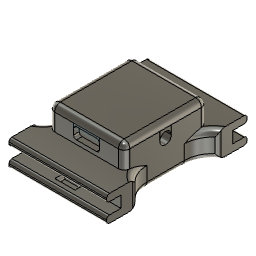
Tremolometer case (Autodesk Fusion 360 design; units mm, degrees)
Autodesk Fusion 360 part; units mm, degrees
sketch "Sketch1" plane through (0, 0, 0) normal (0, 0, 1) x (1, 0, 0)
  line L0 (0, 0) -> (26.2, 0)
  line L1 (26.2, 0) -> (26.2, 28.9)
  line L2 (26.2, 28.9) -> (0, 28.9)
  line L3 (0, 28.9) -> (0, 0)
  dimension "d4" = 26.2
  dimension "d5" = 28.9
  constraint horizontal L0
  constraint vertical L1
  constraint horizontal L2
  constraint vertical L3
  constraint coincident L0.start L3.end
  measures "d4" distance of L0.start L0.end
  measures "d5" distance of L0.start L2.end
extrude "Extrude1" add sketch "Sketch1" along normal blind 15 makes body 1
sketch "Sketch2" plane through (0, 0, 15) normal (0, 0, 1) x (-1, 0, 0)
  line L0 (-4, -24.9) -> (-22.2, -24.9)
  line L1 (-22.2, -24.9) -> (-22.2, -2)
  line L2 (-22.2, -2) -> (-4, -2)
  line L3 (-4, -2) -> (-4, -24.9)
  line L4 (0, -28.9) -> (0, 0)
  line L5 (-26.2, -28.9) -> (0, -28.9)
  line L6 (-26.2, 0) -> (-26.2, -28.9)
  line L7 (0, 0) -> (-26.2, 0)
  dimension "d9" = 4
  dimension "d10" = 4
  dimension "d11" = 4
  dimension "d12" = 2
  constraint horizontal L0
  constraint vertical L1
  constraint horizontal L2
  measures "d9" distance of L3 L4
  measures "d10" distance of L0 L5
  measures "d11" distance of L1 L6
  measures "d12" distance of L2 L7
extrude "Extrude2" cut sketch "Sketch2" against normal blind 6 contours L0 L1 L2 L3 bodies 1
sketch "Sketch4" plane through (0, 0, 0) normal (0, -1, 0) x (1, 0, 0)
  line L0 (0, 0) -> (26.2, 0)
  line L1 (26.2, 0) -> (26.2, 15)
  line L2 (26.2, 15) -> (0, 15)
  line L3 (0, 15) -> (0, 0)
  line L4 (9.6, 10.38) -> (16.6, 10.38)
  line L5 (17.6, 11.38) -> (17.6, 13.38)
  line L6 (16.6, 14.38) -> (9.6, 14.38)
  line L7 (8.6, 13.38) -> (8.6, 11.38)
  arc A0 (9.6, 14.38) -> (8.6, 13.38) centre (9.6, 13.38) ccw
  arc A1 (17.6, 13.38) -> (16.6, 14.38) centre (16.6, 13.38) ccw
  arc A2 (16.6, 10.38) -> (17.6, 11.38) centre (16.6, 11.38) ccw
  arc A3 (8.6, 11.38) -> (9.6, 10.38) centre (9.6, 11.38) ccw
  point P0 (8.6, 10.38)
  point P1 (17.6, 10.38)
  point P2 (8.6, 14.38)
  dimension "d26" = 9
  dimension "d27" = 4
  dimension "d28" = 1
  dimension "d29" = 1
  dimension "d30" = 1
  dimension "d31" = 1
  dimension "d32" = 0.62
  dimension "d33" = 8.6
  constraint horizontal L4
  constraint vertical L5
  constraint horizontal L6
  constraint vertical L7
  constraint coincident P2 L6
  constraint coincident P2 L7
  constraint tangent L6 A0
  constraint tangent L7 A0
  constraint tangent L6 A1
  constraint tangent L5 A1
  constraint coincident P1 L5
  constraint coincident P1 L4
  constraint tangent L5 A2
  constraint tangent L4 A2
  constraint coincident P0 L7
  constraint coincident P0 L4
  constraint tangent L7 A3
  constraint tangent L4 A3
  measures "d26" distance of P0 P1
  measures "d27" distance of P0 P2
  measures "d28" radius of A0
  measures "d29" radius of A1
  measures "d30" radius of A2
  measures "d31" radius of A3
  measures "d32" distance of L2 L6
  measures "d33" distance of L1 L5
extrude "Extrude3" cut sketch "Sketch4" against normal blind 6 contours L4 L5 L6 L7 A0 A1 A2 A3 bodies 1
sketch "Sketch5" plane through (26.2, 0, 0) normal (1, 0, 0) x (0, 1, 0)
  line L0 (0, 0) -> (28.9, 0)
  line L1 (28.9, 0) -> (28.9, 15)
  line L2 (28.9, 15) -> (0, 15)
  line L3 (0, 15) -> (0, 0)
  circle A0 centre (14.45, 12) radius 2
  dimension "d37" = 4
  dimension "d38" = 14.45
  dimension "d39" = 3
  measures "d37" diameter of A0
  measures "d38" distance of L3 A0.centre
  measures "d39" distance of L2 A0.centre
extrude "Extrude4" cut sketch "Sketch5" against normal blind 8.5 contours A0 bodies 1
sketch "Sketch9" plane through (0, 0, 15) normal (0, 0, 1) x (-1, 0, 0)
  line L0 (-22.2, -24.9) -> (-22.2, -2)
  line L1 (-22.2, -2) -> (-4, -2)
  line L2 (-4, -2) -> (-4, -24.9)
  line L3 (-4, -24.9) -> (-22.2, -24.9)
  line L4 (0, -28.9) -> (0, 0)
  line L5 (0, 0) -> (-26.2, 0)
  line L6 (-26.2, 0) -> (-26.2, -28.9)
  line L7 (-26.2, -28.9) -> (0, -28.9)
  line L8 (-2, -26.9) -> (-24.2, -26.9)
  line L9 (-24.2, -26.9) -> (-24.2, -2)
  line L10 (-24.2, -2) -> (-2, -2)
  line L11 (-2, -2) -> (-2, -26.9)
  dimension "d71" = 2
  dimension "d72" = 2
  dimension "d73" = 2
  dimension "d74" = 2
  constraint horizontal L8
  constraint vertical L9
  constraint horizontal L10
  constraint vertical L11
  measures "d71" distance of L5 L10
  measures "d72" distance of L6 L9
  measures "d73" distance of L4 L11
  measures "d74" distance of L7 L8
extrude "Extrude8" add sketch "Sketch9" along normal blind 1 contours L0 L2 L3 L8 L9 L10 L11 bodies 1
extrude "Extrude9" add 1 faces at (10.0667, 0.6667, 15) along direction (0, 0, 1) blind 2 separate body on bodies 1 makes body 2
sketch "Sketch10" plane through (0, 26.9, 0) normal (0, -1, 0) x (1, 0, 0)
  line L0 (2, 15) -> (24.2, 15)
  line L1 (24.2, 15) -> (24.2, 17)
  line L2 (24.2, 17) -> (2, 17)
  line L3 (2, 17) -> (2, 15)
  line L4 (2, 17) -> (26.2, 17)
  line L5 (26.2, 17) -> (26.2, 16)
  line L6 (26.2, 16) -> (2, 16)
  line L7 (2, 16) -> (2, 17)
  dimension "d82" = 24.2
  dimension "d83" = 1
  constraint horizontal L4
  constraint vertical L5
  constraint horizontal L6
  constraint vertical L7
  constraint coincident L2.end L3.start
  measures "d82" distance of L2.end L4.end
  measures "d83" distance of L2.end L6.end
extrude "Extrude10" add sketch "Sketch10" along normal blind 26.9 contours L1 L4 L5 L6 bodies 2
sketch "Sketch19" plane through (0, 0, 0) normal (0, -1, 0) x (1, 0, 0)
  line L0 (16.6, 10.38) -> (9.6, 10.38)
  arc A0 (8.6, 11.38) -> (9.6, 10.38) centre (9.6, 11.38) ccw
  line L1 (8.6, 11.38) -> (8.6, 13.38)
  arc A1 (9.6, 14.38) -> (8.6, 13.38) centre (9.6, 13.38) ccw
  line L2 (9.6, 14.38) -> (16.6, 14.38)
  arc A2 (17.6, 13.38) -> (16.6, 14.38) centre (16.6, 13.38) ccw
  line L3 (17.6, 13.38) -> (17.6, 11.38)
  arc A3 (16.6, 10.38) -> (17.6, 11.38) centre (16.6, 11.38) ccw
  line L4 (0, 0) -> (26.2, 0)
  line L5 (26.2, 0) -> (26.2, 15)
  line L6 (26.2, 15) -> (0, 15)
  line L7 (0, 15) -> (0, 0)
  line L8 (0, 0) -> (26.2, 0)
  line L9 (26.2, 0) -> (26.2, 9)
  line L10 (26.2, 9) -> (0, 9)
  line L11 (0, 9) -> (0, 0)
  dimension "d170" = 26.2
  dimension "d171" = 9
  constraint horizontal L8
  constraint vertical L9
  constraint horizontal L10
  constraint vertical L11
  constraint coincident L4.start L7.end
  measures "d170" distance of L4.start L4.end
  measures "d171" distance of L4.start L10.end
extrude "Extrude19" add sketch "Sketch19" along normal blind 10 contours L4 L5 L7 L8 L9 L10 L11 bodies 1
sketch "Sketch20" plane through (26.2, 0, 0) normal (1, 0, 0) x (0, 1, 0)
  circle A0 centre (14.45, 12) radius 2
  line L0 (-10, 0) -> (28.9, 0)
  line L1 (28.9, 0) -> (28.9, 15)
  line L2 (28.9, 15) -> (0, 15)
  line L3 (0, 15) -> (0, 9)
  line L4 (0, 9) -> (-10, 9)
  line L5 (-10, 9) -> (-10, 0)
  line L6 (-10, 9) -> (0, 9)
  line L7 (0, 9) -> (0, 0)
  line L8 (0, 0) -> (-10, 0)
  line L9 (-10, 0) -> (-10, 9)
  dimension "d174" = 10
  dimension "d175" = 9
  constraint horizontal L6
  constraint vertical L7
  constraint horizontal L8
  constraint vertical L9
  constraint coincident L4.end L5.start
  measures "d174" distance of L4.end L3.end
  measures "d175" distance of L4.end L0.start
extrude "Extrude20" add sketch "Sketch20" along normal blind 3.9 contours L0 L4 L5 L6 L7 L8 L9 bodies 1
sketch "Sketch21" plane through (0, 0, 0) normal (-1, 0, 0) x (0, -1, 0)
  line L0 (-28.9, 0) -> (10, 0)
  line L1 (10, 0) -> (10, 9)
  line L2 (10, 9) -> (0, 9)
  line L3 (0, 9) -> (0, 15)
  line L4 (0, 15) -> (-28.9, 15)
  line L5 (-28.9, 15) -> (-28.9, 0)
  line L6 (10, 9) -> (0, 9)
  line L7 (0, 9) -> (0, 0)
  line L8 (0, 0) -> (10, 0)
  line L9 (10, 0) -> (10, 9)
  dimension "d178" = 10
  dimension "d179" = 9
  constraint horizontal L6
  constraint vertical L7
  constraint horizontal L8
  constraint vertical L9
  constraint coincident L1.end L2.start
  measures "d178" distance of L1.end L2.end
  measures "d179" distance of L1.end L0.end
extrude "Extrude21" add sketch "Sketch21" along normal blind 3.9 contours L0 L1 L2 L6 L7 L8 L9 bodies 1
sketch "Sketch22" plane through (0, -10, 0) normal (0, -1, 0) x (1, 0, 0)
  line L0 (-3.9, 0) -> (30.1, 0)
  line L1 (30.1, 0) -> (30.1, 9)
  line L2 (30.1, 9) -> (-3.9, 9)
  line L3 (-3.9, 9) -> (-3.9, 0)
  line L4 (-3.9, 6.5) -> (30.1, 6.5)
  line L5 (30.1, 6.5) -> (30.1, 2.5)
  line L6 (30.1, 2.5) -> (-3.9, 2.5)
  line L7 (-3.9, 2.5) -> (-3.9, 6.5)
  dimension "d182" = 34
  dimension "d183" = 4
  dimension "d184" = 2.5
  constraint horizontal L4
  constraint vertical L5
  constraint horizontal L6
  constraint vertical L7
  constraint coincident L3 L4.start
  measures "d182" distance of L4.start L4.end
  measures "d183" distance of L4.start L6.end
  measures "d184" distance of L2 L4
extrude "Extrude22" cut sketch "Sketch22" against normal blind 5 contours L1 L3 L4 L5 L6 L7 bodies 1
sketch "Sketch23" plane through (0, 0, 6.5) normal (0, 0, -1) x (1, 0, 0)
  line L0 (30.1, 10) -> (-3.9, 10)
  line L1 (-3.9, 10) -> (-3.9, 5)
  line L2 (-3.9, 5) -> (30.1, 5)
  line L3 (30.1, 5) -> (30.1, 10)
  line L4 (10.6, 5) -> (15.6, 5)
  line L5 (15.6, 5) -> (15.6, 7.5)
  line L6 (15.6, 7.5) -> (10.6, 7.5)
  line L7 (10.6, 7.5) -> (10.6, 5)
  dimension "d190" = 5
  dimension "d191" = 2.5
  dimension "d192" = 14.5
  constraint horizontal L4
  constraint vertical L5
  constraint horizontal L6
  constraint vertical L7
  constraint coincident L2 L4.start
  measures "d190" distance of L4.start L4.end
  measures "d191" distance of L4.start L6.end
  measures "d192" distance of L1 L7
extrude "Extrude23" add sketch "Sketch23" along normal blind 1 contours L2 L4 L5 L6 L7 bodies 1
sketch "Sketch24" plane through (0, 0, 2.5) normal (0, 0, 1) x (-1, 0, 0)
  line L0 (3.9, 10) -> (-30.1, 10)
  line L1 (-30.1, 10) -> (-30.1, 5)
  line L2 (-30.1, 5) -> (3.9, 5)
  line L3 (3.9, 5) -> (3.9, 10)
  line L4 (-10.6, 5) -> (-15.6, 5)
  line L5 (-15.6, 5) -> (-15.6, 7.5)
  line L6 (-15.6, 7.5) -> (-10.6, 7.5)
  line L7 (-10.6, 7.5) -> (-10.6, 5)
  dimension "d195" = 5
  dimension "d196" = 2.5
  dimension "d197" = 14.5
  constraint horizontal L4
  constraint vertical L5
  constraint horizontal L6
  constraint vertical L7
  constraint coincident L2 L4.start
  measures "d195" distance of L4.start L4.end
  measures "d196" distance of L4.start L6.end
  measures "d197" distance of L3 L7
extrude "Extrude24" cut sketch "Sketch24" against normal blind 1 contours L2 L4 L5 L6 L7 bodies 1
sketch "Sketch25" plane through (0, 28.9, 0) normal (0, 1, 0) x (-1, 0, 0)
  line L0 (-26.2, 0) -> (0, 0)
  line L1 (0, 0) -> (0, 15)
  line L2 (0, 15) -> (-26.2, 15)
  line L3 (-26.2, 15) -> (-26.2, 0)
  line L4 (-26.2, 0) -> (0, 0)
  line L5 (0, 0) -> (0, 9)
  line L6 (0, 9) -> (-26.2, 9)
  line L7 (-26.2, 9) -> (-26.2, 0)
  dimension "d200" = 26.2
  dimension "d201" = 9
  constraint horizontal L4
  constraint vertical L5
  constraint horizontal L6
  constraint vertical L7
  constraint coincident L0.start L3.end
  measures "d200" distance of L0.start L0.end
  measures "d201" distance of L0.start L6.end
extrude "Extrude25" add sketch "Sketch25" along normal blind 10 contours L0 L1 L3 L4 L5 L6 L7 bodies 1
sketch "Sketch26" plane through (0, 0, 0) normal (-1, 0, 0) x (0, -1, 0)
  line L0 (0, 0) -> (0, 9)
  line L1 (0, 9) -> (0, 15)
  line L2 (0, 15) -> (-28.9, 15)
  line L3 (-28.9, 15) -> (-28.9, 9)
  line L4 (-28.9, 9) -> (-38.9, 9)
  line L5 (-38.9, 9) -> (-38.9, 0)
  line L6 (-38.9, 0) -> (0, 0)
  line L7 (-38.9, 0) -> (-28.9, 0)
  line L8 (-28.9, 0) -> (-28.9, 9)
  line L9 (-28.9, 9) -> (-38.9, 9)
  line L10 (-38.9, 9) -> (-38.9, 0)
  dimension "d204" = 10
  dimension "d205" = 9
  constraint horizontal L7
  constraint vertical L8
  constraint horizontal L9
  constraint vertical L10
  constraint coincident L5.end L6.start
  measures "d204" distance of L5.end L7.end
  measures "d205" distance of L5.end L4.end
extrude "Extrude26" add sketch "Sketch26" along normal blind 3.9 contours L4 L5 L6 L7 L8 L9 L10 bodies 1
sketch "Sketch27" plane through (26.2, 0, 0) normal (1, 0, 0) x (0, 1, 0)
  line L0 (0, 9) -> (0, 0)
  line L1 (0, 0) -> (38.9, 0)
  line L2 (38.9, 0) -> (38.9, 9)
  line L3 (38.9, 9) -> (28.9, 9)
  line L4 (28.9, 9) -> (28.9, 15)
  line L5 (28.9, 15) -> (0, 15)
  line L6 (0, 15) -> (0, 9)
  circle A0 centre (14.45, 12) radius 2
  line L7 (38.9, 0) -> (28.9, 0)
  line L8 (28.9, 0) -> (28.9, 9)
  line L9 (28.9, 9) -> (38.9, 9)
  line L10 (38.9, 9) -> (38.9, 0)
  dimension "d208" = 10
  dimension "d209" = 9
  constraint horizontal L7
  constraint vertical L8
  constraint horizontal L9
  constraint vertical L10
  constraint coincident L1.end L2.start
  measures "d208" distance of L1.end L7.end
  measures "d209" distance of L1.end L2.end
extrude "Extrude27" add sketch "Sketch27" along normal blind 3.9 contours L1 L2 L3 L7 L8 L9 L10 bodies 1
sketch "Sketch28" plane through (0, 38.9, 0) normal (0, 1, 0) x (-1, 0, 0)
  line L0 (-30.1, 0) -> (3.9, 0)
  line L1 (3.9, 0) -> (3.9, 9)
  line L2 (3.9, 9) -> (-30.1, 9)
  line L3 (-30.1, 9) -> (-30.1, 0)
  line L4 (-30.1, 6.5) -> (3.9, 6.5)
  line L5 (3.9, 6.5) -> (3.9, 2.5)
  line L6 (3.9, 2.5) -> (-30.1, 2.5)
  line L7 (-30.1, 2.5) -> (-30.1, 6.5)
  dimension "d212" = 34
  dimension "d213" = 4
  dimension "d214" = 2.5
  constraint horizontal L4
  constraint vertical L5
  constraint horizontal L6
  constraint vertical L7
  constraint coincident L3 L4.start
  measures "d212" distance of L4.start L4.end
  measures "d213" distance of L4.start L6.end
  measures "d214" distance of L2 L4
extrude "Extrude28" cut sketch "Sketch28" against normal blind 5 contours L1 L3 L4 L5 L6 L7 bodies 1
sketch "Sketch29" plane through (0, 0, 2.5) normal (0, 0, 1) x (-1, 0, 0)
  line L0 (-30.1, -38.9) -> (3.9, -38.9)
  line L1 (3.9, -38.9) -> (3.9, -33.9)
  line L2 (3.9, -33.9) -> (-30.1, -33.9)
  line L3 (-30.1, -33.9) -> (-30.1, -38.9)
  line L4 (-15.6, -33.9) -> (-10.6, -33.9)
  line L5 (-10.6, -33.9) -> (-10.6, -36.4)
  line L6 (-10.6, -36.4) -> (-15.6, -36.4)
  line L7 (-15.6, -36.4) -> (-15.6, -33.9)
  dimension "d217" = 5
  dimension "d218" = 2.5
  dimension "d219" = 14.5
  constraint horizontal L4
  constraint vertical L5
  constraint horizontal L6
  constraint vertical L7
  constraint coincident L2 L4.start
  measures "d217" distance of L4.start L4.end
  measures "d218" distance of L4.start L6.end
  measures "d219" distance of L3 L7
extrude "Extrude29" cut sketch "Sketch29" against normal blind 1 contours L2 L4 L5 L6 L7 bodies 1
sketch "Sketch30" plane through (0, 0, 6.5) normal (0, 0, -1) x (1, 0, 0)
  line L0 (-3.9, -38.9) -> (30.1, -38.9)
  line L1 (30.1, -38.9) -> (30.1, -33.9)
  line L2 (30.1, -33.9) -> (-3.9, -33.9)
  line L3 (-3.9, -33.9) -> (-3.9, -38.9)
  line L4 (15.6, -33.9) -> (10.6, -33.9)
  line L5 (10.6, -33.9) -> (10.6, -36.4)
  line L6 (10.6, -36.4) -> (15.6, -36.4)
  line L7 (15.6, -36.4) -> (15.6, -33.9)
  dimension "d222" = 5
  dimension "d223" = 2.5
  dimension "d224" = 14.5
  constraint horizontal L4
  constraint vertical L5
  constraint horizontal L6
  constraint vertical L7
  constraint coincident L2 L4.start
  measures "d222" distance of L4.start L4.end
  measures "d223" distance of L4.start L6.end
  measures "d224" distance of L3 L5
extrude "Extrude30" add sketch "Sketch30" along normal blind 1 contours L2 L4 L5 L6 L7 bodies 1
fillet "Fillet7" radius 10 1 edges at (26.2, 28.9, 4.5) on bodies 1
fillet "Fillet8" radius 10 1 edges at (26.2, 0, 4.5) on bodies 1
fillet "Fillet9" radius 10 1 edges at (0, 28.9, 4.5) on bodies 1
fillet "Fillet10" radius 10 1 edges at (0, 0, 4.5) on bodies 1
fillet "Fillet11" radius 2 14 edges at (-3.9, 0, 4.5) (-3.9, 28.9, 4.5) (30.1, 28.9, 4.5) (30.1, 0, 4.5) (27.2278, 3.5081, 9) (27.2278, 25.3919, 9) (27.2278, 25.3919, 0) (26.2, 14.45, 0) (27.2278, 3.5081, 0) (-1.0278, 3.5081, 9) (-1.0278, 3.5081, 0) (0, 14.45, 0) (-1.0278, 25.3919, 0) (-1.0278, 25.3919, 9) on bodies 1
fillet "Fillet12" radius 1 2 edges at (13.1, -10, 9) (13.1, -10, 6.5) on bodies 1
fillet "Fillet13" radius 1 2 edges at (13.1, -10, 2.5) (13.1, -10, 0) on bodies 1
fillet "Fillet14" radius 1 4 edges at (13.1, 38.9, 9) (13.1, 38.9, 2.5) (13.1, 38.9, 0) (13.1, 38.9, 6.5) on bodies 1
fillet "Fillet15" radius 2 2 edges at (0, 28.9, 12) (26.2, 28.9, 12) on bodies 1
fillet "Fillet16" radius 2 2 edges at (26.2, 0, 12) (0, 0, 12) on bodies 1
fillet "Fillet17" radius 2 4 edges at (26.2, 28.9, 16) (26.2, 0, 16) (0, 0, 16) (0, 28.9, 16) on bodies 2
fillet "Fillet18" radius 2 8 edges at (0.5858, 28.3142, 17) (0, 14.45, 17) (0.5858, 0.5858, 17) (13.1, 0, 17) (25.6142, 0.5858, 17) (26.2, 14.45, 17) (25.6142, 28.3142, 17) (13.1, 28.9, 17) on bodies 2
fillet "Fillet19" radius 1 3 edges at (10.6, -6.25, 5.5) (10.6, -6.25, 2.5) (15.6, -6.25, 2.5) on bodies 1
fillet "Fillet20" radius 1 1 edges at (15.6, -6.25, 5.5) on bodies 1
fillet "Fillet21" radius 1 3 edges at (15.6, 35.15, 2.5) (10.6, 35.15, 2.5) (10.6, 35.15, 5.5) on bodies 1
fillet "Fillet22" radius 1 1 edges at (15.6, 35.15, 5.5) on bodies 1
sketch "Sketch31" plane through (0, 0, 0) normal (0, -1, 0) x (1, 0, 0)
  line L0 (16.6, 10.38) -> (9.6, 10.38)
  arc A0 (8.6, 11.38) -> (9.6, 10.38) centre (9.6, 11.38) ccw
  line L1 (8.6, 11.38) -> (8.6, 13.38)
  arc A1 (9.6, 14.38) -> (8.6, 13.38) centre (9.6, 13.38) ccw
  line L2 (9.6, 14.38) -> (16.6, 14.38)
  arc A2 (17.6, 13.38) -> (16.6, 14.38) centre (16.6, 13.38) ccw
  line L3 (17.6, 13.38) -> (17.6, 11.38)
  arc A3 (16.6, 10.38) -> (17.6, 11.38) centre (16.6, 11.38) ccw
  line L4 (2, 15) -> (2, 9)
  line L5 (2, 9) -> (24.2, 9)
  line L6 (24.2, 9) -> (24.2, 15)
  line L7 (24.2, 15) -> (2, 15)
  line L8 (8.6, 13.38) -> (17.6, 13.38)
  line L9 (17.6, 13.38) -> (17.6, 23.38)
  line L10 (17.6, 23.38) -> (8.6, 23.38)
  line L11 (8.6, 23.38) -> (8.6, 13.38)
  dimension "d264" = 9
  dimension "d265" = 10
  constraint horizontal L8
  constraint vertical L9
  constraint horizontal L10
  constraint vertical L11
  constraint coincident L1.end A1.end
  measures "d264" distance of L1.end A2.start
  measures "d265" distance of L1.end L10.end
extrude "Extrude31" cut sketch "Sketch31" against normal blind 6 contours A1 L2 A2 L8 | A1 L2 A2 L7 L9 L11 | L7 L9 L10 L11 bodies 1
sketch "Sketch32" plane through (26.2, 0, 0) normal (1, 0, 0) x (0, 1, 0)
  circle A0 centre (14.45, 12) radius 2
  line L0 (2, 15) -> (2, 8.9641)
  spline S0 degree 3 poles (2, 8.9641) (4.0056, 8.7679) (6.1227, 7.8056) (7.924, 7) knots 1.512675 1.512675 1.512675 1.512675 2.104633 2.104633 2.104633 2.104633
  line L1 (7.924, 7) -> (7.924, 2)
  line L2 (7.924, 2) -> (20.976, 2)
  line L3 (20.976, 2) -> (20.976, 7)
  spline S1 degree 3 poles (20.976, 7) (22.7773, 7.8056) (24.8944, 8.7679) (26.9, 8.9641) knots 0 0 0 0 0.591958 0.591958 0.591958 0.591958
  line L4 (26.9, 8.9641) -> (26.9, 15)
  line L5 (26.9, 15) -> (2, 15)
  line L6 (12.45, 12) -> (16.45, 12)
  line L7 (16.45, 12) -> (16.45, 22)
  line L8 (16.45, 22) -> (12.45, 22)
  line L9 (12.45, 22) -> (12.45, 12)
  dimension "d268" = 4
  dimension "d269" = 10
  constraint horizontal L6
  constraint vertical L7
  constraint horizontal L8
  constraint vertical L9
  constraint coincident A0 L6.start
  measures "d268" distance of L6.start L6.end
  measures "d269" distance of L6.start L8.end
extrude "Extrude32" cut sketch "Sketch32" against normal blind 5 contours A0 L6 | A0 L5 L7 L9 | L5 L7 L8 L9 picked at (14.8435, 12.8171) bodies 1
sketch "Sketch33" plane through (0, 0, 15) normal (0, 0, -1) x (1, 0, 0)
  line L0 (2, -26.9) -> (2, -2)
  line L1 (2, -2) -> (24.2, -2)
  line L2 (24.2, -2) -> (24.2, -26.9)
  line L3 (24.2, -26.9) -> (2, -26.9)
  arc A0 (0, -26.9) -> (2, -28.9) centre (2, -26.9) ccw
  line L4 (2, -28.9) -> (24.2, -28.9)
  arc A1 (24.2, -28.9) -> (26.2, -26.9) centre (24.2, -26.9) ccw
  line L5 (26.2, -26.9) -> (26.2, -2)
  arc A2 (26.2, -2) -> (24.2, 0) centre (24.2, -2) ccw
  line L6 (24.2, 0) -> (2, 0)
  arc A3 (2, 0) -> (0, -2) centre (2, -2) ccw
  line L7 (0, -2) -> (0, -26.9)
  line L8 (8.6, 0) -> (17.6, 0)
  line L9 (17.6, 0) -> (17.6, -4)
  line L10 (17.6, -4) -> (8.6, -4)
  line L11 (8.6, -4) -> (8.6, 0)
  dimension "d272" = 9
  dimension "d273" = 4
  constraint horizontal L8
  constraint vertical L9
  constraint horizontal L10
  constraint vertical L11
  constraint coincident L6 L8.start
  measures "d272" distance of L8.start L8.end
  measures "d273" distance of L8.start L10.end
extrude "Extrude33" add sketch "Sketch33" against normal blind 1 contours L1 L9 L10 L11 bodies 2
sketch "Sketch34" plane through (0, 0, 15) normal (0, 0, -1) x (1, 0, 0)
  line L0 (2, -26.9) -> (2, -2)
  line L1 (2, -2) -> (8.6, -2)
  line L2 (8.6, -2) -> (8.6, -4)
  line L3 (8.6, -4) -> (17.6, -4)
  line L4 (17.6, -4) -> (17.6, -2)
  line L5 (17.6, -2) -> (24.2, -2)
  line L6 (24.2, -2) -> (24.2, -26.9)
  line L7 (24.2, -26.9) -> (2, -26.9)
  arc A0 (0, -26.9) -> (2, -28.9) centre (2, -26.9) ccw
  line L8 (2, -28.9) -> (24.2, -28.9)
  arc A1 (24.2, -28.9) -> (26.2, -26.9) centre (24.2, -26.9) ccw
  line L9 (26.2, -26.9) -> (26.2, -2)
  arc A2 (26.2, -2) -> (24.2, 0) centre (24.2, -2) ccw
  line L10 (24.2, 0) -> (2, 0)
  arc A3 (2, 0) -> (0, -2) centre (2, -2) ccw
  line L11 (0, -2) -> (0, -26.9)
  line L12 (8.6, -4) -> (17.6, -4)
  line L13 (17.6, -4) -> (17.6, 0)
  line L14 (17.6, 0) -> (8.6, 0)
  line L15 (8.6, 0) -> (8.6, -4)
  constraint horizontal L12
  constraint vertical L13
  constraint horizontal L14
  constraint vertical L15
  constraint coincident L10 L13.end
  constraint coincident L2.end L3.start
extrude "Extrude34" add sketch "Sketch34" along normal blind 1.62 contours L2 L3 L4 L10 L12 L13 L14 L15 bodies 2
sketch "Sketch35" plane through (0, 0, 0) normal (0, -1, 0) x (1, 0, 0)
  line L0 (17.6, 15) -> (8.6, 15)
  line L1 (8.6, 15) -> (8.6, 13.38)
  line L2 (8.6, 13.38) -> (17.6, 13.38)
  line L3 (17.6, 13.38) -> (17.6, 15)
sketch "Sketch36" plane through (0, 0, 0) normal (0, -1, 0) x (1, 0, 0)
  line L0 (8.6, 13.4) -> (17.6, 13.4)
  line L1 (17.6, 13.4) -> (17.6, 13.4)
  line L2 (16.6, 14.4) -> (9.6, 14.4)
  line L3 (8.6, 13.4) -> (8.6, 13.4)
  arc A0 (9.6, 14.4) -> (8.6, 13.4) centre (9.6, 13.4) ccw
  arc A1 (17.6, 13.4) -> (16.6, 14.4) centre (16.6, 13.4) ccw
  point P0 (8.6, 14.4)
  dimension "d278" = 9
  dimension "d279" = 1
  dimension "d280" = 1
  dimension "d281" = 1
  constraint horizontal L0
  constraint horizontal L2
  constraint coincident P0 L2
  constraint coincident P0 L3
  constraint tangent L2 A0
  constraint tangent L2 A1
  measures "d278" distance of L0.start L0.end
  measures "d279" distance of L0.start P0
  measures "d280" radius of A0
  measures "d281" radius of A1
extrude "Extrude35" cut sketch "Sketch36" against normal blind 10 bodies 2
extrude "Extrude36" cut 1 faces at (11.6, 2, 13.38) along direction (0, 0, 1) blind 0.1 on bodies 2 bodies 2
sketch "Sketch41" plane through (0, 0, 15) normal (0, 0, -1) x (1, 0, 0)
  line L0 (8.6, -2) -> (8.6, 0)
  line L1 (8.6, 0) -> (2, 0)
  arc A0 (2, 0) -> (0, -2) centre (2, -2) ccw
  line L2 (0, -2) -> (0, -26.9)
  arc A1 (0, -26.9) -> (2, -28.9) centre (2, -26.9) ccw
  line L3 (2, -28.9) -> (24.2, -28.9)
  arc A2 (24.2, -28.9) -> (26.2, -26.9) centre (24.2, -26.9) ccw
  line L4 (26.2, -26.9) -> (26.2, -2)
  arc A3 (26.2, -2) -> (24.2, 0) centre (24.2, -2) ccw
  line L5 (24.2, 0) -> (17.6, 0)
  line L6 (17.6, 0) -> (17.6, -2)
  line L7 (17.6, -2) -> (24.2, -2)
  line L8 (24.2, -2) -> (24.2, -26.9)
  line L9 (24.2, -26.9) -> (2, -26.9)
  line L10 (2, -26.9) -> (2, -2)
  line L11 (2, -2) -> (8.6, -2)
  line L12 (26.2, -12.4516) -> (22.2, -12.4516)
  line L13 (22.2, -12.4516) -> (22.2, -16.4516)
  line L14 (22.2, -16.4516) -> (26.2, -16.4516)
  line L15 (26.2, -16.4516) -> (26.2, -12.4516)
  dimension "d301" = 4
  dimension "d302" = 4
  constraint horizontal L12
  constraint vertical L13
  constraint horizontal L14
  constraint vertical L15
  constraint coincident L4 L12.start
  measures "d301" distance of L12.start L12.end
  measures "d302" distance of L12.start L14.end
extrude "Extrude42" add sketch "Sketch41" against normal blind 1 contours L8 L12 L13 L14 bodies 2
sketch "Sketch42" plane through (0, 0, 15) normal (0, 0, -1) x (1, 0, 0)
  line L0 (8.6, -2) -> (8.6, 0)
  line L1 (8.6, 0) -> (2, 0)
  arc A0 (2, 0) -> (0, -2) centre (2, -2) ccw
  line L2 (0, -2) -> (0, -26.9)
  arc A1 (0, -26.9) -> (2, -28.9) centre (2, -26.9) ccw
  line L3 (2, -28.9) -> (24.2, -28.9)
  arc A2 (24.2, -28.9) -> (26.2, -26.9) centre (24.2, -26.9) ccw
  line L4 (26.2, -26.9) -> (26.2, -2)
  arc A3 (26.2, -2) -> (24.2, 0) centre (24.2, -2) ccw
  line L5 (24.2, 0) -> (17.6, 0)
  line L6 (17.6, 0) -> (17.6, -2)
  line L7 (17.6, -2) -> (24.2, -2)
  line L8 (24.2, -2) -> (24.2, -12.4516)
  line L9 (24.2, -12.4516) -> (22.2, -12.4516)
  line L10 (22.2, -12.4516) -> (22.2, -16.4516)
  line L11 (22.2, -16.4516) -> (24.2, -16.4516)
  line L12 (24.2, -16.4516) -> (24.2, -26.9)
  line L13 (24.2, -26.9) -> (2, -26.9)
  line L14 (2, -26.9) -> (2, -2)
  line L15 (2, -2) -> (8.6, -2)
  line L16 (22.2, -12.4516) -> (26.2, -12.4516)
  line L17 (26.2, -12.4516) -> (26.2, -16.4516)
  line L18 (26.2, -16.4516) -> (22.2, -16.4516)
  line L19 (22.2, -16.4516) -> (22.2, -12.4516)
  dimension "d305" = 4
  dimension "d306" = 4
  constraint horizontal L16
  constraint vertical L17
  constraint horizontal L18
  constraint vertical L19
  constraint coincident L9.end L10.start
  measures "d305" distance of L9.end L16.end
  measures "d306" distance of L9.end L10.end
extrude "Extrude43" add sketch "Sketch42" along normal blind 3 contours L4 L9 L10 L11 L16 L17 L18 L19 bodies 2
sketch "Sketch43" plane through (26.2, 0, 0) normal (1, 0, 0) x (0, 1, 0)
  line L0 (16.4516, 15) -> (12.4516, 15)
  line L1 (12.4516, 15) -> (12.4516, 12)
  line L2 (12.4516, 12) -> (16.4516, 12)
  line L3 (16.4516, 12) -> (16.4516, 15)
  circle A0 centre (14.4516, 12) radius 2.05
  dimension "d309" = 4.1
  constraint midpoint L2 A0.centre
  measures "d309" diameter of A0
extrude "Extrude44" cut sketch "Sketch43" against normal blind 10 contours L1 L2 L3 A0 picked at (14.4516, 12.6833) bodies 2
extrude "Extrude45" cut 1 faces at (16.8, 26.9, 16.3333) along direction (0, -1, 0) blind 24.9 on bodies 2 bodies 2
sketch "Sketch44" plane through (0, 26.9, 0) normal (0, -1, 0) x (1, 0, 0)
  line L0 (2, 15) -> (24.2, 15)
  line L1 (24.2, 15) -> (24.2, 17)
  line L2 (24.2, 17) -> (2, 17)
  line L3 (2, 17) -> (2, 15)
  line L4 (24.2, 17) -> (2, 17)
  line L5 (2, 17) -> (2, 16)
  line L6 (2, 16) -> (24.2, 16)
  line L7 (24.2, 16) -> (24.2, 17)
  dimension "d316" = 22.2
  dimension "d317" = 1
  constraint horizontal L4
  constraint vertical L5
  constraint horizontal L6
  constraint vertical L7
  constraint coincident L1.end L2.start
  measures "d316" distance of L1.end L2.end
  measures "d317" distance of L1.end L6.end
extrude "Extrude47" add sketch "Sketch44" along normal blind 24.9 contours L1 L2 L3 L4 L5 L6 L7 bodies 2
extrude "Extrude48" add 1 faces at (14.6, 3.3333, 15) along direction (0, 0, 1) blind 1 on bodies 2 bodies 2
extrude "Extrude49" add 1 faces at (23.5333, 13.7849, 15) along direction (0, 0, 1) blind 1 on bodies 2 bodies 2
equation "Tiny_Length = 22.9 mm - USB_Length_Outside_Tiny"
equation "Tiny_Width = 18.2 mm"
equation "Tiny_Height = 6 mm"
equation "d4 = Tiny_Width + ( Tiny_Wall_Width * 2 )"
equation "d5 = Tiny_Length + ( Tiny_Wall_Width * 2 )"
equation "Tiny_Wall_Width = 4 mm"
equation "d7 = Wristband_Extension_Height + Tiny_Height"
equation "d9 = Tiny_Wall_Width"
equation "d10 = Tiny_Wall_Width"
equation "d11 = Tiny_Wall_Width"
equation "d12 = Tiny_Wall_Width - USB_Length_Outside_Tiny"
equation "d13 = -Tiny_Height"
equation "USB_Corner_Radius = 1 mm"
equation "USB_Length = 9 mm"
equation "USB_Height_Without_Corner = 2 mm"
equation "d26 = USB_Length"
equation "d27 = USB_Height_Without_Corner + 2 * USB_Corner_Radius"
equation "d28 = USB_Corner_Radius"
equation "d29 = USB_Corner_Radius"
equation "d30 = USB_Corner_Radius"
equation "d31 = USB_Corner_Radius"
equation "d32 = Tiny_Height - Tiny_Wall_Width - ( 0.5 * 2.76 ) * 1 mm"
equation "d33 = ( Tiny_Width + ( 2 * Tiny_Wall_Width ) ) / 2 - USB_Length / 2"
equation "Tiny_Cable_Hole_Radius = 4 mm"
equation "d37 = Tiny_Cable_Hole_Radius"
equation "d38 = ( Tiny_Length + 2 * Tiny_Wall_Width ) * 0.5"
equation "d39 = Tiny_Height / 2"
equation "Snap_In_Length = 10 mm"
equation "Snap_In_Height = 3 mm"
equation "Snap_In_Depth = 3 mm"
equation "Snap_In_Margin = 0.5 mm"
equation "Mini_Snap_In_Length = 4 mm"
equation "Mini_Snap_In_Height = 2 mm"
equation "Track_Width = 1 mm"
equation "d71 = Track_Width + Track_Margin"
equation "d72 = Track_Width + Track_Margin"
equation "d73 = Track_Width + Track_Margin"
equation "d74 = Track_Width + Track_Margin"
equation "Track_Height = 1 mm"
equation "d76 = Track_Height"
equation "d79 = Top_Height"
equation "Top_Height = 2 mm"
equation "d82 = Tiny_Width + 2 * Tiny_Wall_Width - 2 * Track_Width"
equation "d83 = Track_Height"
equation "d84 = Tiny_Wall_Width * 2 + Tiny_Length - 2 * Track_Width"
equation "Fillet_Amount = 2 mm"
equation "Stand_Size = 2 mm"
equation "Stand_Height = 1 mm"
equation "Wristband_Length = 34 mm"
equation "Wristband_Height = 3 mm"
equation "USB_Length_Outside_Tiny = 2 mm"
equation "Tiny_Corner_To_Attachment = 1 mm"
equation "Tiny_Attachment_Hole_Radius = 1 mm"
equation "Tiny_Attachment_Height = 2 mm"
equation "WristBand_Extension_Single_Side_Length = ( Wristband_Length - ( Tiny_Width + 2 * Tiny_Wall_Width ) ) / 2"
equation "Wristband_Extension_Depth = 10 mm"
equation "Wristband_Extension_Height = 3 * Wristband_Height"
equation "d170 = 2 * Tiny_Wall_Width + Tiny_Width"
equation "d171 = Wristband_Extension_Height"
equation "d172 = Wristband_Extension_Depth"
equation "d174 = Wristband_Extension_Depth"
equation "d175 = Wristband_Extension_Height"
equation "d176 = WristBand_Extension_Single_Side_Length"
equation "d178 = Wristband_Extension_Depth"
equation "d179 = Wristband_Extension_Height"
equation "d180 = WristBand_Extension_Single_Side_Length"
equation "d182 = Wristband_Length"
equation "d183 = Wristband_Height + 1 mm"
equation "d184 = ( ( Wristband_Extension_Height - 1 mm ) - Wristband_Height ) / 2"
equation "Wristband_Depth = 5 mm"
equation "d186 = -Wristband_Depth"
equation "Wristband_Lock_Width = 5 mm"
equation "Wristband_lock_Height = 1 mm"
equation "d190 = Wristband_Lock_Width"
equation "d191 = Wristband_Depth / 2"
equation "d192 = ( Wristband_Length - Wristband_Lock_Width ) / 2"
equation "d193 = Wristband_lock_Height"
equation "d195 = Wristband_Lock_Width"
equation "d196 = Wristband_Depth / 2"
equation "d197 = ( Wristband_Length - Wristband_Lock_Width ) / 2"
equation "d198 = -Wristband_lock_Height"
equation "d200 = 2 * Tiny_Wall_Width + Tiny_Width"
equation "d201 = Wristband_Extension_Height"
equation "d202 = Wristband_Extension_Depth"
equation "d204 = Wristband_Extension_Depth"
equation "d205 = Wristband_Extension_Height"
equation "d206 = WristBand_Extension_Single_Side_Length"
equation "d208 = Wristband_Extension_Depth"
equation "d209 = Wristband_Extension_Height"
equation "d210 = WristBand_Extension_Single_Side_Length"
equation "d212 = Wristband_Length"
equation "d213 = Wristband_Height + 1 mm"
equation "d214 = ( Wristband_Extension_Height - 1 mm - Wristband_Height ) / 2"
equation "d215 = -Wristband_Depth"
equation "d217 = Wristband_Lock_Width"
equation "d218 = Wristband_Depth / 2"
equation "d219 = ( Wristband_Length - Wristband_Lock_Width ) / 2"
equation "d220 = -Wristband_lock_Height"
equation "d222 = Wristband_Lock_Width"
equation "d223 = Wristband_Depth / 2"
equation "d224 = ( Wristband_Length - Wristband_Lock_Width ) / 2"
equation "d225 = Wristband_lock_Height"
equation "Tiny_Side_Support_Depth = 10 mm"
equation "d229 = Tiny_Side_Support_Depth"
equation "d231 = Tiny_Side_Support_Depth"
equation "d233 = Tiny_Side_Support_Depth"
equation "d235 = Tiny_Side_Support_Depth"
equation "d237 = Fillet_Amount"
equation "Small_Fillet_Amount = Fillet_Amount / 2"
equation "d240 = Small_Fillet_Amount"
equation "d242 = Small_Fillet_Amount"
equation "d244 = Small_Fillet_Amount"
equation "d246 = Fillet_Amount"
equation "d248 = Fillet_Amount"
equation "d250 = Fillet_Amount"
equation "d252 = Fillet_Amount"
equation "Wristband_Lock_Fillet = 1 mm"
equation "d255 = Wristband_Lock_Fillet"
equation "d257 = Wristband_Lock_Fillet"
equation "d259 = Wristband_Lock_Fillet"
equation "d261 = Wristband_Lock_Fillet"
equation "Track_Margin = 1 mm"
equation "Tiny_Bottom_Height_Modifier = 5 mm"
equation "d264 = USB_Length"
equation "d268 = Tiny_Cable_Hole_Radius"
equation "d272 = USB_Length"
equation "d273 = Tiny_Wall_Width"
equation "d276 = 3.62 mm - USB_Height_Without_Corner"
equation "d278 = USB_Length"
equation "d279 = USB_Corner_Radius"
equation "d280 = USB_Corner_Radius"
equation "d281 = USB_Corner_Radius"
equation "d301 = Tiny_Wall_Width"
equation "d302 = Tiny_Cable_Hole_Radius"
equation "d305 = Tiny_Wall_Width"
equation "d306 = Tiny_Cable_Hole_Radius"
equation "d307 = Tiny_Height / 2"
equation "d309 = Tiny_Cable_Hole_Radius + 0.1 mm"
equation "d312 = Tiny_Length + Tiny_Wall_Width"
equation "d316 = Tiny_Width + Tiny_Wall_Width"
equation "d317 = Track_Margin"
equation "d318 = Tiny_Length + Tiny_Wall_Width"
